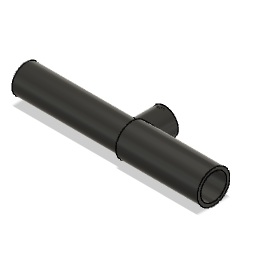
Assemblage bravabot (Autodesk Fusion 360 archive; units mm, degrees)
design "Canon"
Autodesk Fusion 360 part; units mm, degrees
(part 1 of 2)
sketch "Sketch1" plane through (0, 0, 0) normal (0, 0, 1) x (1, 0, 0)
  circle A0 centre (0, 0) radius 16.5
  circle A1 centre (0, 0) radius 15.5
  line L0 (-25, -5) -> (25, -5)
  line L1 (25, -5) -> (25, 5)
  line L2 (25, 5) -> (-25, 5)
  line L3 (-25, 5) -> (-25, -5)
  line L4 (-25, -5) -> (25, 5) construction
  line L5 (25, -5) -> (-25, 5) construction
  line L6 (-5, 25) -> (5, 25)
  line L7 (5, 25) -> (5, -25)
  line L8 (5, -25) -> (-5, -25)
  line L9 (-5, -25) -> (-5, 25)
  line L10 (-5, 25) -> (5, -25) construction
  line L11 (5, 25) -> (-5, -25) construction
  circle A2 centre (0, 4) radius 1
  circle A3 centre (0, -4) radius 1
  circle A4 centre (-3, 0) radius 1
  circle A5 centre (3, 0) radius 1
  dimension "d1" = 33
  dimension "d15" = 31
  dimension "d18" = 50
  dimension "d19" = 10
  dimension "d20" = 10
  dimension "d21" = 50
  dimension "d22" = 2
  dimension "d23" = 2
  dimension "d25" = 2
  dimension "d26" = 4
  dimension "d27" = 8
  dimension "d28" = 2
  dimension "d29" = 3
  dimension "d30" = 6
  constraint coincident A0.centre A1.centre
  constraint horizontal L0
  constraint perpendicular L0 L1
  constraint parallel L0 L2
  constraint parallel L1 L3
  constraint coincident L4 A0.centre
  constraint coincident L5 A0.centre
  constraint horizontal L6
  constraint perpendicular L6 L7
  constraint parallel L6 L8
  constraint parallel L7 L9
  constraint coincident L10 A0.centre
  constraint coincident L11 A0.centre
  measures "d1" diameter of A0
  measures "d15" diameter of A1
  measures "d18" distance of L1.end L2.end
  measures "d19" distance of L0.end L1.end
  measures "d20" distance of L7.end L8.end
  measures "d21" distance of L6.end L7.end
  measures "d22" diameter of A2
  measures "d23" diameter of A3
  measures "d25" diameter of A4
  measures "d26" distance of A0.centre A3.centre
  measures "d27" distance of A2.centre A3.centre
  measures "d28" diameter of A5
  measures "d29" distance of A0.centre A5.centre
  measures "d30" distance of A4.centre A5.centre
extrude "Extrude1" add sketch "Sketch1" along normal blind 37 contours A0 A1 L0 L2 | A0 A1 L2 L7 | A0 A1 L0 L7 | A0 A1 L7 L9 | A1 L2 L7 | A1 L0 L2 L7 | A0 A1 L7 L9 | A1 L0 L7 | A0 A1 L2 L9 | A1 L2 L7 L9 | A2 | A3 | L0 L2 L7 L9 | A0 A1 L0 L9 | A1 L0 L7 L9 | A0 A1 L0 L2 | A1 L2 L9 | A1 L0 L9 | A1 L0 L2 L9 | A4 | A5
sketch "Sketch2" plane through (0, 0, 0) normal (1, 0, 0) x (0, 0, -1)
  circle A0 centre (-39.9957, 0.4126) radius 20
  circle A1 centre (-39.9957, 0.4126) radius 17.5
  circle A2 centre (-39.9957, 0.4126) radius 16
  dimension "d4" = 40
  dimension "d7" = 35
  dimension "d10" = 32
  constraint concentric A0 A1
  constraint concentric A1 A2
  measures "d4" diameter of A0
  measures "d7" diameter of A1
  measures "d10" diameter of A2
extrude "Extrude2" add sketch "Sketch2" along normal blind 100 contours A0 | A1 | A2
extrude "Extrude3" add sketch "Sketch2" against normal blind 130 contours A1 | A2
extrude "Extrude4" cut sketch "Sketch2" along normal blind 140 and the other way blind 90 contours A2
extrude "Extrude5" cut sketch "Sketch1" along normal blind 40 contours A1 L2 L7 | A1 L0 L2 L7 | A1 L0 L7 | A1 L2 L7 L9 | A2 | A3 | L0 L2 L7 L9 | A1 L0 L7 L9 | A1 L2 L9 | A1 L0 L9 | A1 L0 L2 L9 | A4 | A5
extrude "Extrude6" add sketch "Sketch1" along normal blind 2 from surface at 3 contours A1 L0 L2 L7 | A1 L2 L7 L9 | L0 L2 L7 L9 | A1 L0 L7 L9 | A1 L0 L2 L9

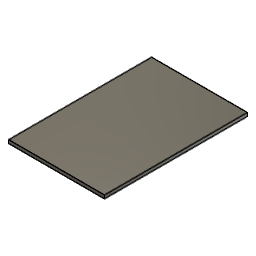
design "Raspberry"
Autodesk Fusion 360 part; units mm, degrees
sketch "Sketch1" plane through (0, 0, 0) normal (0, 1, 0) x (1, 0, 0)
  line L0 (-23.8395, 24.7876) -> (33.1605, 24.7876)
  line L1 (33.1605, 24.7876) -> (33.1605, -60.2124)
  line L2 (33.1605, -60.2124) -> (-23.8395, -60.2124)
  line L3 (-23.8395, -60.2124) -> (-23.8395, 24.7876)
  dimension "d1" = 57
  dimension "d2" = 85
  constraint horizontal L0
  constraint vertical L1
  constraint horizontal L2
  constraint vertical L3
  measures "d1" distance of L0.start L0.end
  measures "d2" distance of L0.start L2.end
extrude "Extrude1" add sketch "Sketch1" along normal blind 2

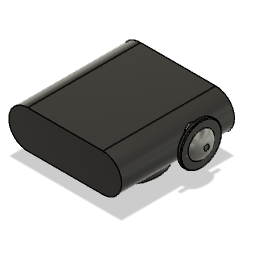
design "tete"
Autodesk Fusion 360 part; units mm, degrees
sketch "Sketch1" plane through (0, 0, 0) normal (0, 0, 1) x (1, 0, 0)
  line L0 (50, 50) -> (0, 50)
  line L1 (0, 50) -> (0, 48)
  arc A0 (50, 0) -> (50, 50) centre (50, 25) ccw
  line L2 (0, 48) -> (48, 48)
  arc A1 (50, 2.0871) -> (48, 48) centre (48, 25) ccw
  arc A2 (-48, 48) -> (-50, 2.0871) centre (-48, 25) ccw
  line L3 (0, 50) -> (0, 48)
  line L4 (-50, 50) -> (0, 50)
  arc A3 (-50, 50) -> (-50, 0) centre (-50, 25) ccw
  line L5 (0, 48) -> (-48, 48)
  line L6 (100, -50) -> (-100, -50)
  line L7 (-100, -50) -> (-100, 100)
  line L8 (-100, 100) -> (100, 100)
  line L9 (100, 100) -> (100, -50)
  line L10 (30.6667, 48) -> (33.3333, 50) construction
  line L11 (-50, 2.0871) -> (-50, 0)
  line L12 (50, 2.0871) -> (50, 0)
  line L13 (-30.6667, 48) -> (-33.3333, 50) construction
  line L14 (-50, 2.0871) -> (50, 2.0871)
  dimension "d1" = 50
  dimension "d2" = 50
  dimension "d8" = 46
  dimension "d9" = 200
  dimension "d10" = 150
  constraint horizontal L0
  constraint vertical L1
  constraint tangent L0 A0
  constraint symmetric A0.start L1 A3.end
  constraint symmetric L0.start L1 L4.start
  constraint symmetric L0.end L1 L3.start
  constraint symmetric L1 A0 A3
  constraint symmetric L1 L2.end A2.start
  constraint symmetric L1 A1 A2
  constraint horizontal L6
  constraint perpendicular L6 L7
  constraint parallel L6 L8
  constraint parallel L7 L9
  constraint vertical L11
  constraint parallel L7 L12
  constraint coincident L2 L10.start
  constraint coincident L5 L13.start
  constraint coincident L0 L10.end
  constraint coincident L4 L13.end
  measures "d1" distance of origin A0.start
  measures "d2" distance of origin L0.end
  measures "d8" diameter of A1
  measures "d9" distance of L7.end L8.end
  measures "d10" distance of L6.end L7.end
extrude "Extrude1" add sketch "Sketch1" along normal blind 146 contours L0 L1 A0 L2 A1 L3 L12 | L1 A2 L3 L4 A3 L5 L11 makes body 1
sketch "Sketch2" plane through (0, 50, 0) normal (0, 1, 0) x (-1, 0, 0)
  line L0 (-50, 0) -> (50, 0)
  line L1 (50, 0) -> (50, 146)
  line L2 (50, 146) -> (-50, 146)
  line L3 (-50, 146) -> (-50, 0)
  line L4 (75, 0) -> (-75, 0)
  line L5 (-75, 0) -> (-75, -2)
  line L6 (-75, -2) -> (75, -2)
  line L7 (75, -2) -> (75, 0)
  line L8 (75, 146) -> (-75, 146)
  line L9 (-75, 146) -> (-75, 148)
  line L10 (-75, 148) -> (75, 148)
  line L11 (75, 148) -> (75, 146)
  dimension "d13" = 150
  dimension "d14" = 2
  dimension "d15" = 150
  dimension "d16" = 2
  constraint horizontal L4
  constraint vertical L5
  constraint horizontal L6
  constraint vertical L7
  constraint horizontal L8
  constraint vertical L9
  constraint horizontal L10
  constraint vertical L11
  measures "d13" distance of L4.start L4.end
  measures "d14" distance of L4.start L6.end
  measures "d15" distance of L8.start L8.end
  measures "d16" distance of L8.start L10.end
extrude "Extrude2" add sketch "Sketch2" against normal blind 70 contours L0 L4 L5 L6 L7 | L2 L8 L9 L10 L11 bodies 1
extrude "Extrude3" cut sketch "Sketch1" along normal blind 150 and the other way blind 50 bodies 1
sketch "Sketch3" plane through (0, 2.0871, 0) normal (0, -1, 0) x (1, 0, 0)
  line L0 (50, 148) -> (-50, 148)
  line L1 (-50, 148) -> (-50, 146)
  line L2 (-50, 146) -> (50, 146)
  line L3 (50, 146) -> (50, 148)
  circle A0 centre (0, 73) radius 48
  circle A1 centre (0, 73) radius 46
  line L4 (-50, 148) -> (50, 148)
  line L5 (50, 148) -> (50, -2)
  line L6 (50, -2) -> (-50, -2)
  line L7 (-50, -2) -> (-50, 148)
  line L8 (-5, 15) -> (5, 15)
  line L9 (5, 15) -> (5, 131)
  line L10 (5, 131) -> (-5, 131)
  line L11 (-5, 131) -> (-5, 15)
  line L12 (-5, 15) -> (5, 131) construction
  line L13 (5, 15) -> (-5, 131) construction
  line L14 (58, 78) -> (-58, 78)
  line L15 (-58, 78) -> (-58, 68)
  line L16 (-58, 68) -> (58, 68)
  line L17 (58, 68) -> (58, 78)
  line L18 (58, 78) -> (-58, 68) construction
  line L19 (-58, 78) -> (58, 68) construction
  circle A2 centre (0, 67) radius 1
  circle A3 centre (4, 73) radius 1
  circle A4 centre (-4, 73) radius 1
  circle A5 centre (0, 79) radius 1
  point P0 (0, 73)
  point P1 (0, 73)
  dimension "d23" = 96
  dimension "d24" = 75
  dimension "d25" = 92
  dimension "d33" = 116
  dimension "d34" = 10
  dimension "d35" = 2
  dimension "d36" = 2
  dimension "d37" = 2
  dimension "d38" = 2
  dimension "d39" = 12
  dimension "d40" = 6
  dimension "d41" = 4
  dimension "d42" = 8
  constraint concentric A0 A1
  constraint horizontal L4
  constraint vertical L5
  constraint horizontal L6
  constraint vertical L7
  constraint coincident L0.end L1.start
  constraint horizontal L8
  constraint perpendicular L8 L9
  constraint parallel L8 L10
  constraint parallel L9 L11
  constraint coincident L12 P1
  constraint coincident L13 P1
  constraint coincident P1 P0
  constraint horizontal L14
  constraint perpendicular L14 L15
  constraint parallel L14 L16
  constraint parallel L15 L17
  constraint coincident L18 P1
  constraint coincident L19 P1
  measures "d23" diameter of A0
  measures "d24" distance of L0 P1
  measures "d25" diameter of A1
  measures "d33" distance of L15.end L16.end
  measures "d34" distance of L14.end L15.end
  measures "d35" diameter of A2
  measures "d36" diameter of A3
  measures "d37" diameter of A4
  measures "d38" diameter of A5
  measures "d39" distance of A2.centre A5.centre
  measures "d40" distance of P1 A2.centre
  measures "d41" distance of P1 A4.centre
  measures "d42" distance of A3.centre A4.centre
extrude "Extrude4" add sketch "Sketch3" along normal blind 2 contours L0 L1 L2 L3 L4 L5 L7 | L2 A0 L5 L7 L9 L10 L11 L14 | A0 L5 L14 L16 | A0 L7 L14 L16 | A0 L5 L6 L7 L8 L9 L11 L16 | A0 L9 L10 L11 | A0 L8 L9 L11 bodies 1
extrude "Extrude5" add sketch "Sketch3" along normal blind 20 contours A0 A1 L9 L14 | A0 A1 L14 L16 | A0 A1 L14 L16 | A0 A1 L11 L14 | A0 A1 L9 L16 | A0 A1 L9 L11 | A0 A1 L11 L16 | A0 A1 L9 L11 bodies 1
sketch "Sketch4" plane through (0, 0, -2) normal (0, 0, -1) x (-1, 0, 0)
  arc A0 (-50, 50) -> (-50, 0) centre (-50, 25) ccw
  line L0 (-50, 0) -> (-50, 0.0871)
  line L1 (-50, 0.0871) -> (50, 0.0871)
  line L2 (50, 0.0871) -> (50, 0)
  arc A1 (50, 0) -> (50, 50) centre (50, 25) ccw
  line L3 (50, 50) -> (-50, 50)
  circle A2 centre (0, 25) radius 17.5
  line L4 (20, 20) -> (-20, 20)
  line L5 (-20, 20) -> (-20, 30)
  line L6 (-20, 30) -> (20, 30)
  line L7 (20, 30) -> (20, 20)
  line L8 (20, 20) -> (-20, 30) construction
  line L9 (-20, 20) -> (20, 30) construction
  line L10 (-6.6445, 5) -> (6.6445, 5)
  line L11 (6.6445, 5) -> (6.6445, 45)
  line L12 (6.6445, 45) -> (-6.6445, 45)
  line L13 (-6.6445, 45) -> (-6.6445, 5)
  line L14 (-6.6445, 5) -> (6.6445, 45) construction
  line L15 (6.6445, 5) -> (-6.6445, 45) construction
  line L16 (13.5, 19) -> (-13.5, 19)
  line L17 (-13.5, 19) -> (-13.5, 31)
  line L18 (-13.5, 31) -> (13.5, 31)
  line L19 (13.5, 31) -> (13.5, 19)
  line L20 (13.5, 19) -> (-13.5, 31) construction
  line L21 (-13.5, 19) -> (13.5, 31) construction
  line L22 (14.5, 18) -> (-14.5, 18)
  line L23 (-14.5, 18) -> (-14.5, 32)
  line L24 (-14.5, 32) -> (14.5, 32)
  line L25 (14.5, 32) -> (14.5, 18)
  line L26 (14.5, 18) -> (-14.5, 32) construction
  line L27 (-14.5, 18) -> (14.5, 32) construction
  point P0 (0, 25)
  point P1 (0, 25)
  point P2 (0, 25)
  point P3 (0, 25)
  dimension "d30" = 35
  dimension "d45" = 40
  dimension "d46" = 10
  dimension "d47" = 40
  dimension "d48" = 27
  dimension "d49" = 12
  dimension "d50" = 29
  dimension "d51" = 14
  constraint horizontal L4
  constraint perpendicular L4 L5
  constraint parallel L4 L6
  constraint parallel L5 L7
  constraint coincident L8 P3
  constraint coincident L9 P3
  constraint coincident P3 P2
  constraint horizontal L10
  constraint perpendicular L10 L11
  constraint parallel L10 L12
  constraint parallel L11 L13
  constraint coincident L14 P3
  constraint coincident L15 P3
  constraint horizontal L16
  constraint perpendicular L16 L17
  constraint parallel L16 L18
  constraint parallel L17 L19
  constraint coincident L20 P3
  constraint coincident L21 P3
  constraint horizontal L22
  constraint perpendicular L22 L23
  constraint parallel L22 L24
  constraint parallel L23 L25
  constraint coincident L26 P3
  constraint coincident L27 P3
  measures "d30" diameter of A2
  measures "d45" distance of L5.end L6.end
  measures "d46" distance of L4.end L5.end
  measures "d47" distance of L10.end L11.end
  measures "d48" distance of L17.end L18.end
  measures "d49" distance of L16.end L17.end
  measures "d50" distance of L23.end L24.end
  measures "d51" distance of L22.end L23.end
extrude "Extrude6" cut sketch "Sketch4" against normal blind 20 contours A2 L4 L6 L25 | A2 L6 L11 L24 L25 | A2 L4 L11 L22 L25 | A2 L11 L13 L24 | L4 L6 L19 L25 | L6 L11 L18 L19 L24 L25 | A2 L11 L13 L22 | L4 L11 L16 L19 L22 L25 | A2 L6 L13 L23 L24 | L11 L13 L18 L24 | L4 L6 L11 L19 | L6 L11 L18 L19 | A2 L4 L13 L22 L23 | L11 L13 L16 L22 | L4 L11 L16 L19 | A2 L4 L6 L23 | L6 L13 L17 L18 L23 L24 | L6 L11 L13 L18 | L4 L6 L11 L13 | L4 L13 L16 L17 L22 L23 | L4 L11 L13 L16 | L4 L6 L17 L23 | L6 L13 L17 L18 | L4 L6 L13 L17 | L4 L13 L16 L17 bodies 1
extrude "Extrude7" add sketch "Sketch3" along normal blind 3 contours A1 L9 L14 L16 | A1 L11 L14 L16 | A1 L9 L11 L14 | L9 L11 L14 L16 | A1 L9 L11 L16 bodies 1
extrude "Extrude8" add sketch "Sketch4" against normal blind 9 contours A2 L4 L6 L7 | A2 L11 L12 L13 | A2 L10 L11 L13 | A2 L4 L5 L6 bodies 1
extrude "Extrude9" add sketch "Sketch4" along normal blind 2 and the other way blind 15 separate body contours L4 L6 L19 L25 | L6 L11 L18 L19 L24 L25 | L4 L11 L16 L19 L22 L25 | L11 L13 L18 L24 | L11 L13 L16 L22 | L6 L13 L17 L18 L23 L24 | L4 L13 L16 L17 L22 L23 | L4 L6 L17 L23 makes body 2
extrude "Extrude10" add sketch "Sketch4" against normal blind 3 from surface at -6 separate body contours A2 L4 L6 L25 | A2 L11 L13 L24 | A2 L11 L13 L22 | A2 L4 L6 L23 makes body 3 at (0, 14.5, 4) makes body 4 at (0, 35.5, 4) makes body 5 at (16.9923, 20.8154, 6) makes body 6 at (-17.4184, 23.3124, 5)
ref_plane "WorkPlane1" through (75, 0, 0) normal (1, 0, 0) x (0, 1, 0)
sketch "Sketch6" plane through (75, 0, 0) normal (1, 0, 0) x (0, 0, -1)
  circle A0 centre (-50, 25) radius 17.5
  circle A1 centre (-50, 25) radius 27.5
  dimension "d62" = 35
  dimension "d63" = 55
  constraint concentric A0 A1
  measures "d62" diameter of A0
  measures "d63" diameter of A1
extrude "Extrude11" add sketch "Sketch6" along normal blind 15 and the other way blind 10 contours A0 bodies 1 6 5 4 3 2
extrude "Extrude12" add sketch "Sketch6" along normal blind 5 from surface at 3 bodies 1 2 3 6 5 4
fillet "Fillet1" radius 17.5 1 edges at (90, 18.6717, 66.3157) on bodies 1
fillet "Fillet2" radius 1 2 edges at (83, 15.0556, 75.639) (78, 15.0556, 75.639) on bodies 1

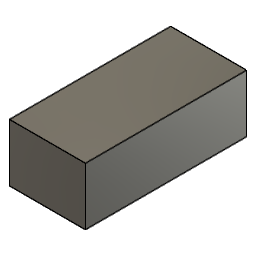
design "Batterie"
Autodesk Fusion 360 part; units mm, degrees
sketch "Sketch1" plane through (0, 0, 0) normal (0, 1, 0) x (1, 0, 0)
  line L0 (-8, 7) -> (-41, 7)
  line L1 (-41, 7) -> (-41, -63)
  line L2 (-41, -63) -> (-8, -63)
  line L3 (-8, -63) -> (-8, 7)
  dimension "d1" = 33
  dimension "d2" = 70
  constraint horizontal L0
  constraint vertical L1
  constraint horizontal L2
  constraint vertical L3
  measures "d1" distance of L0.start L0.end
  measures "d2" distance of L0.start L2.end
extrude "Extrude1" add sketch "Sketch1" along normal blind 25

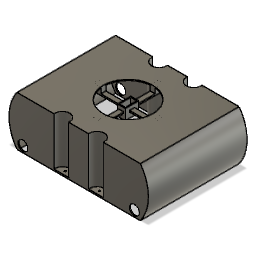
design "Carter BravaBot"
Autodesk Fusion 360 part; units mm, degrees
sketch "Sketch1" plane through (0, 0, 0) normal (0, 0, 1) x (1, 0, 0)
  line L0 (0, 0) -> (-125, 0)
  line L1 (-125, 100) -> (0, 100)
  line L2 (0, 100) -> (0, 0)
  arc A0 (-125, 100) -> (-125, 0) centre (-56.2614, 50) ccw
  arc A1 (-124.4112, 98) -> (-123, 0) centre (-54.2614, 50) ccw
  line L3 (0, 98) -> (-124.4112, 98)
  line L4 (-175, 98) -> (-175, -10)
  line L5 (-175, -10) -> (191.1619, -10)
  line L6 (191.1619, -10) -> (191.1619, 126.0853)
  line L7 (191.1619, 126.0853) -> (-175, 126.0853)
  line L8 (-175, 126.0853) -> (-175, 98)
  line L9 (0, 98) -> (124.4112, 98)
  line L10 (125, 100) -> (0, 100)
  arc A2 (123, 0) -> (124.4112, 98) centre (54.2614, 50) ccw
  arc A3 (125, 0) -> (125, 100) centre (56.2614, 50) ccw
  line L11 (0, 0) -> (125, 0)
  circle A4 centre (113, 12.5) radius 10
  circle A5 centre (-113, 12.5) radius 10
  dimension "d1" = 125
  dimension "d2" = 100
  dimension "d3" = 85
  dimension "d4" = 85
  dimension "d6" = 2
  dimension "d7" = 2
  dimension "d44" = 20
  dimension "d45" = 12
  dimension "d46" = 12.5
  constraint horizontal L0
  constraint horizontal L1
  constraint vertical L2
  constraint coincident L0.start L2.end
  constraint coincident L0 A1.end
  constraint coincident L2 L3.start
  constraint perpendicular L2 L3
  constraint perpendicular L3 L4
  constraint perpendicular L4 L5
  constraint perpendicular L5 L6
  constraint perpendicular L6 L7
  constraint perpendicular L3 L8
  constraint symmetric L0.start L2 L11.start
  constraint symmetric L0.end L2 A3.start
  constraint symmetric L1.start L2 L10.start
  constraint symmetric L1.end L2 L10.end
  constraint symmetric L2 A0 A3
  constraint symmetric L2 A1.end A2.start
  constraint symmetric L2 A1 A2
  constraint symmetric L2 L3.start L9.start
  constraint symmetric L2 A1.start L9.end
  constraint symmetric L2 A4 A5
  measures "d1" distance of L0.start L0.end
  measures "d2" distance of L0.start L1.end
  measures "d3" radius of A0
  measures "d4" radius of A1
  measures "d6" distance of L0.end A1.end
  measures "d7" distance of L1 L3
  measures "d44" diameter of A4
  measures "d45" horizontal distance of A3.start A4.centre
  measures "d46" distance of L11 A4.centre
extrude "Extrude1" add sketch "Sketch1" along normal blind 196 contours L0 L1 L2 A0 A1 L3 | L2 L9 L10 A2 A3 L11 makes body 1
sketch "Sketch2" plane through (0, 100, 0) normal (0, 1, 0) x (-1, 0, 0)
  line L0 (-125, 0) -> (125, 0)
  line L1 (125, 0) -> (125, 196)
  line L2 (125, 196) -> (-125, 196)
  line L3 (-125, 196) -> (-125, 0)
  line L4 (56.5763, 0) -> (165.4437, 0)
  line L5 (165.4437, 0) -> (165.4437, -2)
  line L6 (165.4437, -2) -> (56.5763, -2)
  line L7 (56.5763, -2.1497) -> (56.5763, -2)
  line L8 (27.1632, 196) -> (155, 196)
  line L9 (155, 196) -> (155, 198)
  line L10 (155, 198) -> (27.1632, 198)
  line L11 (27.1632, 196) -> (-160, 196)
  line L12 (-160, 196) -> (-160, 198)
  line L13 (-160, 198) -> (27.1632, 198)
  line L14 (56.5763, 0) -> (-160, 0)
  line L15 (-160, 0) -> (-160, -2)
  line L16 (-160, -2) -> (56.5763, -2)
  line L17 (56.5763, -2) -> (56.5763, 0)
  circle A0 centre (-35, 196) radius 15
  circle A1 centre (-35, 196) radius 17
  circle A2 centre (35, 196) radius 15
  circle A3 centre (35, 196) radius 17
  circle A4 centre (-35, 0) radius 17
  circle A5 centre (-35, 0) radius 15
  circle A6 centre (35, 0) radius 17
  circle A7 centre (35, 0) radius 15
  circle A8 centre (-35, 6) radius 2
  circle A9 centre (35, 6) radius 2
  line L18 (-50, 0) -> (-50, 25)
  line L19 (20, 0) -> (20, 24.2158)
  circle A10 centre (35, 190) radius 2
  circle A11 centre (-35, 190) radius 2
  circle A12 centre (0, 98) radius 50
  line L20 (65, 103) -> (65, 93)
  line L21 (-65, 93) -> (-65, 103)
  line L22 (-5, 33) -> (5, 33)
  line L23 (5, 163) -> (-5, 163)
  line L24 (-6, 109.5) -> (6, 109.5)
  line L25 (6, 86.5) -> (-6, 86.5)
  line L26 (-8, 93) -> (-65, 93)
  line L27 (65, 93) -> (8, 93)
  line L28 (5, 33) -> (5, 84.5)
  line L29 (5, 111.5) -> (5, 163)
  line L30 (65, 103) -> (8, 98.6154) construction
  line L31 (-8, 97.3846) -> (-65, 93) construction
  line L32 (-65, 103) -> (-8, 98.6154) construction
  line L33 (8, 97.3846) -> (65, 93) construction
  line L34 (-125, 98) -> (-8, 98)
  line L35 (8, 98) -> (125, 98)
  line L36 (-5, 33) -> (-1.0385, 84.5) construction
  line L37 (1.0385, 111.5) -> (5, 163) construction
  line L38 (5, 33) -> (1.0385, 84.5) construction
  line L39 (-1.0385, 111.5) -> (-5, 163) construction
  line L40 (-65, 103) -> (-8, 103)
  line L41 (8, 103) -> (65, 103)
  line L42 (-5, 84.5) -> (-5, 33)
  line L43 (-5, 163) -> (-5, 111.5)
  line L44 (6, 109.5) -> (6, 98)
  line L45 (6, 97.5385) -> (6, 86.5)
  line L46 (-6, 86.5) -> (-6, 98.4615)
  line L47 (-6, 103) -> (-6, 109.5)
  line L48 (-6, 103) -> (-6, 98.4615)
  line L49 (-8, 84.5) -> (8, 84.5)
  line L50 (8, 84.5) -> (8, 111.5)
  line L51 (8, 111.5) -> (-8, 111.5)
  line L52 (-8, 111.5) -> (-8, 84.5)
  line L53 (6, 98) -> (6, 97.5385)
  point P0 (0, 98)
  point P1 (0, 98)
  point P2 (0, 98)
  point P3 (0, 98)
  dimension "d10" = 2
  dimension "d11" = 2
  dimension "d12" = 2
  dimension "d15" = 2
  dimension "d22" = 30
  dimension "d23" = 34
  dimension "d24" = 30
  dimension "d25" = 34
  dimension "d26" = 90
  dimension "d27" = 90
  dimension "d35" = 4
  dimension "d36" = 4
  dimension "d37" = 15
  dimension "d38" = 15
  dimension "d39" = 6
  dimension "d40" = 6
  dimension "d41" = 100
  dimension "d55" = 130
  dimension "d56" = 10
  dimension "d57" = 10
  dimension "d58" = 130
  dimension "d59" = 12
  dimension "d60" = 23
  dimension "d61" = 16
  dimension "d62" = 27
  constraint perpendicular L4 L5
  constraint parallel L4 L6
  constraint perpendicular L1 L4
  constraint coincident L0 L4.start
  constraint vertical L7
  constraint horizontal L8
  constraint vertical L9
  constraint horizontal L10
  constraint coincident L2 L8.start
  constraint horizontal L11
  constraint vertical L12
  constraint horizontal L13
  constraint horizontal L14
  constraint vertical L15
  constraint horizontal L16
  constraint vertical L17
  constraint concentric A0 A1
  constraint concentric A2 A3
  constraint midpoint L3 L34.start
  constraint midpoint L1 L35.end
  constraint coincident L8 A2.centre
  constraint coincident L11 A0.centre
  constraint symmetric A0 A5 L34
  constraint symmetric A1 A4 L34
  constraint symmetric A2 A7 L34
  constraint symmetric A3 A6 L34
  constraint coincident A5 L18.start
  constraint coincident L14 L18.start
  constraint tangent A5 L18
  constraint coincident A7 L19.start
  constraint coincident L14 L19.start
  constraint tangent A7 L19
  constraint symmetric A8 A11 L34
  constraint symmetric A9 A10 L34
  constraint horizontal L40
  constraint perpendicular L20 L40
  constraint parallel L27 L40
  constraint parallel L20 L21
  constraint coincident P3 L32
  constraint coincident P3 L30
  constraint coincident P3 P2
  constraint horizontal L22
  constraint perpendicular L22 L28
  constraint parallel L22 L23
  constraint parallel L28 L43
  constraint coincident P3 L36
  constraint coincident P3 L38
  constraint horizontal L24
  constraint perpendicular L24 L44
  constraint parallel L24 L25
  constraint parallel L44 L46
  constraint collinear L26 L27
  constraint collinear L30 L31
  constraint collinear L32 L33
  constraint collinear L34 L35
  constraint collinear L36 L37
  constraint collinear L38 L39
  constraint collinear L40 L41
  constraint collinear L42 L43
  constraint coincident L47.start L46
  constraint coincident L45.start L44
  constraint collinear L44 L45
  constraint collinear L46 L47
  constraint horizontal L49
  constraint perpendicular L49 L50
  constraint parallel L49 L51
  constraint parallel L50 L52
  constraint coincident L49 L28.end
  constraint coincident L50 L27.end
  constraint coincident L50 L35.start
  constraint coincident L50 L33.start
  constraint coincident L50 L30.end
  constraint coincident L50 L41.start
  constraint coincident L52 L34.end
  constraint coincident L52 L32.end
  constraint coincident L52 L31.start
  constraint coincident L52 L26.start
  constraint coincident L49 L42.start
  constraint coincident L49 L36.end
  constraint coincident L49 L38.end
  constraint coincident L52 L40.end
  constraint coincident L51 L43.end
  constraint coincident L51 L29.start
  constraint coincident L51 L37.start
  constraint coincident L51 L39.start
  measures "d10" distance of L8 L10
  measures "d11" distance of L11 L13
  measures "d12" distance of L4 L6
  measures "d15" distance of L4.start L6.end
  measures "d22" diameter of A0
  measures "d23" diameter of A1
  measures "d24" diameter of A2
  measures "d25" diameter of A3
  measures "d26" distance of L3 A0.centre
  measures "d27" distance of L1 A2.centre
  measures "d35" diameter of A8
  measures "d36" diameter of A9
  measures "d37" distance of A8.centre L18
  measures "d38" distance of A9.centre L19
  measures "d39" distance of L14 A8.centre
  measures "d40" distance of L14 A9.centre
  measures "d41" diameter of A12
  measures "d55" distance of L20.end L21.start
  measures "d56" distance of L27 L40
  measures "d57" distance of L23.start L23.end
  measures "d58" distance of L22.end L23.start
  measures "d59" distance of L25.start L25.end
  measures "d60" distance of L24.end L25.start
  measures "d61" distance of L50.end L51.end
  measures "d62" distance of L49.end L50.end
extrude "Extrude2" add sketch "Sketch2" against normal blind 100 contours L0 L14 L16 A4 A5 | L0 L14 L16 A5 | L0 L14 L16 A4 A5 | L0 L14 L15 L16 A4 | L0 L14 L16 A4 A6 | L0 L14 L16 A6 A7 | L0 L14 L16 A7 | L2 L11 L12 L13 A1 | L0 L14 L16 A6 A7 | L0 L14 L16 L17 A6 | L2 L11 L13 A0 A1 | L0 L4 L5 L6 L17 | L2 L11 L13 A0 | L2 L11 L13 A1 A3 | L2 L11 L13 A0 A1 | L2 L11 L13 A2 A3 | L2 L8 L10 L11 L13 A2 | L2 L8 L9 L10 A3 | L2 L8 L10 A2 A3 bodies 1
extrude "Extrude3" cut sketch "Sketch1" along normal blind 270 and the other way blind 120 contours L4 L5 L6 L7 L8 bodies 1
extrude "Extrude4" cut sketch "Sketch2" against normal blind 120 contours L0 L14 A5 | L0 L14 L16 A5 | L0 L14 A7 | L0 L14 L16 A7 | L2 L11 L13 A0 | L2 L11 A0 | L2 L8 L10 L11 L13 A2 | L2 L8 L11 A2 | A8 | A9 | A10 | A11 bodies 1
extrude "Extrude5" add sketch "Sketch2" against normal blind 100 contours L0 L14 L16 A4 A5 | L0 L14 A4 A5 L18 | L0 L14 A4 L18 | L0 L14 L16 A4 A5 | L0 L14 A6 L19 | L0 L14 L16 A6 A7 | L0 L14 A6 A7 L19 | L0 L14 L16 A6 A7 | L2 L11 L13 A0 A1 | L2 L11 A0 A1 | L2 L11 L13 A0 A1 | L2 L11 L13 A2 A3 | L2 L8 L11 A2 A3 | L2 L8 L10 A2 A3 bodies 1
extrude "Extrude6" add sketch "Sketch2" against normal blind 3 from surface at -97 contours L0 L14 A5 | L0 L14 L16 A5 | L0 L14 A7 | L0 L14 L16 A7 | L2 L11 L13 A0 | L2 L11 A0 | L2 L8 L10 L11 L13 A2 | L2 L8 L11 A2 | A8 | A9 | A10 | A11 bodies 1
extrude "Extrude7" cut sketch "Sketch2" against normal blind 180 contours A12 L26 L34 L52 | A12 L34 L40 L52 | A12 L26 L42 L49 L52 | A12 L40 L43 L51 L52 | L49 L50 L51 L52 | A12 L28 L42 L49 | A12 L29 L43 L51 | A12 L27 L28 L49 L50 | A12 L29 L41 L50 L51 | A12 L27 L35 L50 | A12 L35 L41 L50 | A8 | A9 | A10 | A11 | L24 L25 L44 L45 L46 L47 L48 L53 bodies 1
extrude "Extrude8" cut sketch "Sketch1" along normal blind 250 and the other way blind 25 contours A4 | A5 bodies 1
extrude "Extrude9" add sketch "Sketch2" against normal blind 3 from surface at -12.5 separate body contours A12 L26 L34 L52 | A12 L34 L40 L52 | A12 L28 L42 L49 | A12 L29 L43 L51 | A12 L27 L35 L50 | A12 L35 L41 L50 makes body 2 at (0.5564, 87.5, 123.6574) makes body 3 at (21.9907, 84.5, 98.5564) makes body 4 at (-21.9907, 84.5, 98.5564) makes body 5 at (0.5564, 87.5, 72.3426)
extrude "Extrude10" add sketch "Sketch2" against normal blind 21.5 from surface at -5 contours L49 L50 L51 L52 bodies 2 3 4 5
extrude "Extrude11" add sketch "Sketch2" against normal blind 2 from surface at -24.5 contours L24 L25 L44 L45 L46 L47 L48 L53 bodies 2
extrude "Extrude12" add sketch "Sketch2" against normal blind 15.5 contours A12 L21 L26 L34 | A12 L21 L34 L40 | A12 L22 L28 L42 | A12 L23 L29 L43 | A12 L20 L35 L41 | A12 L20 L27 L35 bodies 1 2
sketch "Sketch3" plane through (0, 0, 86.5) normal (0, 0, 1) x (1, 0, 0)
  line L0 (-6, 75.5) -> (6, 75.5)
  line L1 (6, 75.5) -> (6, 95)
  line L2 (6, 95) -> (-6, 95)
  line L3 (-6, 95) -> (-6, 75.5)
  line L4 (-5, 77) -> (5, 77)
  line L5 (5, 77) -> (5, 84.4286)
  line L6 (5, 84.4286) -> (-5, 84.4286)
  line L7 (-5, 84.4286) -> (-5, 77)
  constraint horizontal L4
  constraint vertical L5
  constraint horizontal L6
  constraint vertical L7
extrude "Extrude13" cut sketch "Sketch3" against normal blind 2 contours L4 L5 L6 L7 bodies 1

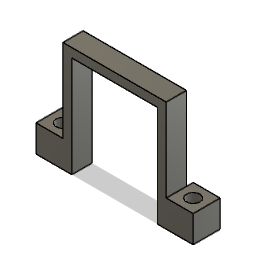
design "fixation moto-réducteur"
Autodesk Fusion 360 part; units mm, degrees
sketch "Sketch1" plane through (0, 0, 0) normal (0, 0, 1) x (1, 0, 0)
  line L0 (0, 0) -> (6, 0)
  line L1 (6, 0) -> (6, 6)
  line L2 (6, 6) -> (0, 6)
  line L3 (0, 6) -> (0, 0)
  line L4 (6, 0) -> (8, 0)
  line L5 (8, 0) -> (8, 24.5)
  line L6 (8, 24.5) -> (6, 24.5)
  line L7 (6, 24.5) -> (6, 0)
  line L8 (6, 24.5) -> (17.5, 24.5)
  line L9 (17.5, 24.5) -> (17.5, 22.5)
  line L10 (17.5, 22.5) -> (6, 22.5)
  line L11 (6, 22.5) -> (6, 24.5)
  line L12 (29, 6) -> (35, 6)
  line L13 (17.5, 22.5) -> (29, 22.5)
  line L14 (29, 0) -> (29, 6)
  line L15 (35, 6) -> (35, 0)
  line L16 (29, 24.5) -> (29, 0)
  line L17 (27, 24.5) -> (29, 24.5)
  line L18 (17.5, 24.5) -> (17.5, 22.5)
  line L19 (29, 22.5) -> (29, 24.5)
  line L20 (35, 0) -> (29, 0)
  line L21 (29, 24.5) -> (17.5, 24.5)
  line L22 (27, 0) -> (27, 24.5)
  line L23 (29, 0) -> (27, 0)
  point P0 (35, 0)
  dimension "d1" = 6
  dimension "d2" = 6
  dimension "d3" = 2
  dimension "d4" = 24.5
  dimension "d5" = 11.5
  dimension "d6" = 2
  constraint horizontal L0
  constraint vertical L1
  constraint horizontal L2
  constraint vertical L3
  constraint coincident L0.start L3.end
  constraint horizontal L4
  constraint vertical L5
  constraint horizontal L6
  constraint vertical L7
  constraint horizontal L8
  constraint vertical L9
  constraint horizontal L10
  constraint vertical L11
  constraint symmetric L0.start L9 L15.end
  constraint symmetric L0.start L9 P0
  constraint symmetric L0.end L9 L14.start
  constraint symmetric L1.end L9 L12.start
  constraint symmetric L2.end L9 L12.end
  constraint symmetric L4.end L9 L22.start
  constraint symmetric L5.end L9 L17.start
  constraint symmetric L6.end L9 L16.start
  constraint symmetric L8.end L9 L18.start
  constraint symmetric L10.start L9 L13.start
  constraint symmetric L10.end L9 L13.end
  measures "d1" distance of L0.start L0.end
  measures "d2" distance of L0.start L2.end
  measures "d3" distance of L0.end L4.end
  measures "d4" distance of L0.end L6.end
  measures "d5" distance of L6.end L8.end
  measures "d6" distance of L6.end L10.end
extrude "Extrude1" add sketch "Sketch1" along normal blind 3 and the other way blind 3 contours L0 L1 L2 L3 L7 | L12 L14 L15 L16 L20 makes body 1 at (31, 6, -1) makes body 2 at (0, 2, 1)
extrude "Extrude2" add sketch "Sketch1" along normal blind 1.5 and the other way blind 1.5 contours L1 L4 L5 L7 L10 | L5 L6 L7 L8 L10 L11 | L5 L8 L9 L10 L18 | L9 L13 L18 L21 L22 | L13 L16 L17 L19 L21 L22 | L13 L14 L16 L22 L23 bodies 1 2
sketch "Sketch3" plane through (0, 6, 0) normal (0, 1, 0) x (-1, 0, 0)
  line L0 (0, -3) -> (0, 3)
  line L1 (0, 3) -> (-6, 3)
  line L2 (-6, 3) -> (-6, 1.5)
  line L3 (-6, 1.5) -> (-6, -1.5)
  line L4 (-6, -1.5) -> (-6, -3)
  line L5 (-6, -3) -> (0, -3)
  circle A0 centre (-3, 0) radius 1.5
  circle A1 centre (-32, 0) radius 1.5
  line L6 (-35, -3) -> (-35, 3)
  line L7 (-29, -3) -> (-35, -3)
  dimension "d16" = 3
  dimension "d17" = 3
  dimension "d18" = 3
  dimension "d19" = 3
  dimension "d20" = 3
  dimension "d21" = 3
  measures "d16" diameter of A0
  measures "d17" diameter of A1
  measures "d18" distance of L5 A0.centre
  measures "d19" distance of L0 A0.centre
  measures "d20" distance of A1.centre L6
  measures "d21" distance of A1.centre L7
extrude "Extrude3" cut sketch "Sketch3" against normal blind 11 contours A0 | A1 bodies 1
extrude "Extrude4" add 1 faces at (27.6667, 9.5, 1.5) along direction (0, 0, 1) up to surface (1.5 mm away) on bodies 1 bodies 1

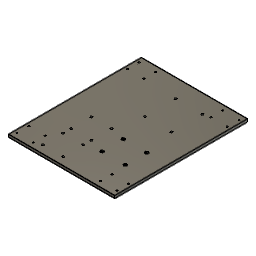
design "base roulante essaie"
Autodesk Fusion 360 part; units mm, degrees
sketch "Sketch1" plane through (0, 0, 0) normal (0, 1, 0) x (1, 0, 0)
  line L0 (0, 0) -> (200, 0)
  line L1 (200, 0) -> (200, 250)
  line L2 (200, 250) -> (0, 250)
  line L3 (0, 250) -> (0, 0)
  circle A0 centre (6, 240) radius 1.5
  circle A1 centre (37, 240) radius 1.5
  line L4 (100, 250) -> (100, 0)
  line L5 (0, 125) -> (200, 125)
  circle A2 centre (163, 240) radius 1.5
  circle A3 centre (194, 240) radius 1.5
  circle A4 centre (6, 10) radius 1.5
  circle A5 centre (163, 10) radius 1.5
  circle A6 centre (37, 10) radius 1.5
  circle A7 centre (194, 10) radius 1.5
  circle A8 centre (6, 218) radius 1.5
  circle A9 centre (37, 218) radius 1.5
  circle A10 centre (163, 218) radius 1.5
  circle A11 centre (194, 218) radius 1.5
  circle A12 centre (37, 32) radius 1.5
  circle A13 centre (6, 32) radius 1.5
  circle A14 centre (194, 32) radius 1.5
  circle A15 centre (163, 32) radius 1.5
  line L6 (34.25, 238.4123) -> (37, 236.8246)
  line L7 (37, 236.8246) -> (39.75, 238.4123)
  line L8 (39.75, 238.4123) -> (39.75, 241.5877)
  line L9 (39.75, 241.5877) -> (37, 243.1754)
  line L10 (37, 243.1754) -> (34.25, 241.5877)
  line L11 (34.25, 241.5877) -> (34.25, 238.4123)
  line L12 (8.75, 238.4123) -> (8.75, 241.5877)
  line L13 (8.75, 241.5877) -> (6, 243.1754)
  line L14 (6, 243.1754) -> (3.25, 241.5877)
  line L15 (3.25, 241.5877) -> (3.25, 238.4123)
  line L16 (3.25, 238.4123) -> (6, 236.8246)
  line L17 (6, 236.8246) -> (8.75, 238.4123)
  line L18 (34.25, 219.5877) -> (34.25, 216.4123)
  line L19 (34.25, 216.4123) -> (37, 214.8246)
  line L20 (37, 214.8246) -> (39.75, 216.4123)
  line L21 (39.75, 216.4123) -> (39.75, 219.5877)
  line L22 (39.75, 219.5877) -> (37, 221.1754)
  line L23 (37, 221.1754) -> (34.25, 219.5877)
  line L24 (3.25, 219.5877) -> (3.25, 216.4123)
  line L25 (3.25, 216.4123) -> (6, 214.8246)
  line L26 (6, 214.8246) -> (8.75, 216.4123)
  line L27 (8.75, 216.4123) -> (8.75, 219.5877)
  line L28 (8.75, 219.5877) -> (6, 221.1754)
  line L29 (6, 221.1754) -> (3.25, 219.5877)
  line L30 (191.25, 238.4123) -> (191.25, 241.5877)
  line L31 (194, 214.8246) -> (191.25, 216.4123)
  line L32 (160.25, 219.5877) -> (163, 221.1754)
  line L33 (163, 214.8246) -> (160.25, 216.4123)
  line L34 (163, 236.8246) -> (160.25, 238.4123)
  line L35 (194, 221.1754) -> (196.75, 219.5877)
  line L36 (191.25, 219.5877) -> (194, 221.1754)
  line L37 (196.75, 219.5877) -> (196.75, 216.4123)
  line L38 (194, 236.8246) -> (191.25, 238.4123)
  line L39 (160.25, 238.4123) -> (160.25, 241.5877)
  line L40 (160.25, 216.4123) -> (160.25, 219.5877)
  line L41 (196.75, 238.4123) -> (194, 236.8246)
  line L42 (196.75, 216.4123) -> (194, 214.8246)
  line L43 (160.25, 241.5877) -> (163, 243.1754)
  line L44 (165.75, 219.5877) -> (165.75, 216.4123)
  line L45 (196.75, 241.5877) -> (196.75, 238.4123)
  line L46 (163, 221.1754) -> (165.75, 219.5877)
  line L47 (165.75, 216.4123) -> (163, 214.8246)
  line L48 (194, 243.1754) -> (196.75, 241.5877)
  line L49 (191.25, 216.4123) -> (191.25, 219.5877)
  line L50 (165.75, 238.4123) -> (163, 236.8246)
  line L51 (191.25, 241.5877) -> (194, 243.1754)
  line L52 (163, 243.1754) -> (165.75, 241.5877)
  line L53 (165.75, 241.5877) -> (165.75, 238.4123)
  line L54 (8.75, 33.5877) -> (8.75, 30.4123)
  line L55 (37, 28.8246) -> (34.25, 30.4123)
  line L56 (34.25, 8.4123) -> (34.25, 11.5877)
  line L57 (37, 35.1754) -> (39.75, 33.5877)
  line L58 (6, 35.1754) -> (8.75, 33.5877)
  line L59 (34.25, 33.5877) -> (37, 35.1754)
  line L60 (37, 6.8246) -> (34.25, 8.4123)
  line L61 (3.25, 8.4123) -> (3.25, 11.5877)
  line L62 (39.75, 11.5877) -> (39.75, 8.4123)
  line L63 (6, 13.1754) -> (8.75, 11.5877)
  line L64 (37, 13.1754) -> (39.75, 11.5877)
  line L65 (39.75, 8.4123) -> (37, 6.8246)
  line L66 (39.75, 30.4123) -> (37, 28.8246)
  line L67 (8.75, 11.5877) -> (8.75, 8.4123)
  line L68 (8.75, 30.4123) -> (6, 28.8246)
  line L69 (34.25, 11.5877) -> (37, 13.1754)
  line L70 (3.25, 30.4123) -> (3.25, 33.5877)
  line L71 (34.25, 30.4123) -> (34.25, 33.5877)
  line L72 (8.75, 8.4123) -> (6, 6.8246)
  line L73 (3.25, 33.5877) -> (6, 35.1754)
  line L74 (6, 6.8246) -> (3.25, 8.4123)
  line L75 (39.75, 33.5877) -> (39.75, 30.4123)
  line L76 (6, 28.8246) -> (3.25, 30.4123)
  line L77 (3.25, 11.5877) -> (6, 13.1754)
  line L78 (191.25, 8.4123) -> (194, 6.8246)
  line L79 (165.75, 11.5877) -> (163, 13.1754)
  line L80 (194, 6.8246) -> (196.75, 8.4123)
  line L81 (165.75, 30.4123) -> (165.75, 33.5877)
  line L82 (163, 28.8246) -> (165.75, 30.4123)
  line L83 (196.75, 11.5877) -> (194, 13.1754)
  line L84 (191.25, 30.4123) -> (194, 28.8246)
  line L85 (194, 13.1754) -> (191.25, 11.5877)
  line L86 (196.75, 33.5877) -> (194, 35.1754)
  line L87 (165.75, 33.5877) -> (163, 35.1754)
  line L88 (194, 35.1754) -> (191.25, 33.5877)
  line L89 (165.75, 8.4123) -> (165.75, 11.5877)
  line L90 (160.25, 11.5877) -> (160.25, 8.4123)
  line L91 (196.75, 30.4123) -> (196.75, 33.5877)
  line L92 (163, 6.8246) -> (165.75, 8.4123)
  line L93 (160.25, 33.5877) -> (160.25, 30.4123)
  line L94 (163, 13.1754) -> (160.25, 11.5877)
  line L95 (191.25, 11.5877) -> (191.25, 8.4123)
  line L96 (196.75, 8.4123) -> (196.75, 11.5877)
  line L97 (160.25, 30.4123) -> (163, 28.8246)
  line L98 (160.25, 8.4123) -> (163, 6.8246)
  line L99 (191.25, 33.5877) -> (191.25, 30.4123)
  line L100 (163, 35.1754) -> (160.25, 33.5877)
  line L101 (194, 28.8246) -> (196.75, 30.4123)
  point P0 (37, 240)
  point P1 (6, 240)
  point P2 (37, 218)
  point P3 (6, 218)
  point P4 (194, 240)
  point P5 (163, 218)
  point P6 (163, 218)
  point P7 (194, 240)
  point P8 (194, 218)
  point P9 (6, 10)
  point P10 (37, 10)
  point P11 (37, 10)
  point P12 (6, 32)
  point P13 (6, 10)
  point P14 (6, 32)
  point P15 (37, 32)
  point P16 (37, 32)
  point P17 (194, 10)
  point P18 (163, 10)
  point P19 (194, 32)
  point P20 (163, 32)
  point P21 (163, 32)
  point P22 (194, 32)
  point P23 (194, 10)
  point P24 (163, 32)
  point P25 (194, 10)
  dimension "d1" = 200
  dimension "d2" = 250
  dimension "d3" = 3
  dimension "d4" = 6
  dimension "d5" = 10
  dimension "d6" = 3
  dimension "d8" = 10
  dimension "d11" = 3
  dimension "d12" = 3
  dimension "d13" = 32
  dimension "d14" = 32
  dimension "d15" = 6
  dimension "d16" = 31
  dimension "d17" = 31
  dimension "d19" = 2.75
  dimension "d20" = 2.75
  dimension "d21" = 2.75
  dimension "d22" = 2.75
  constraint horizontal L0
  constraint vertical L1
  constraint horizontal L2
  constraint vertical L3
  constraint coincident L0.start L3.end
  constraint midpoint L2 L4.start
  constraint midpoint L0 L4.end
  constraint midpoint L3 L5.start
  constraint midpoint L1 L5.end
  constraint symmetric A0 L4 A3
  constraint symmetric A1 L4 A2
  constraint symmetric A0 L5 A4
  constraint symmetric A1 L5 A6
  constraint symmetric L5 A2 A5
  constraint symmetric L5 A3 A7
  constraint symmetric L4 A8 A11
  constraint symmetric L4 A9 A10
  constraint symmetric L5 A8 A13
  constraint symmetric L5 A9 A12
  constraint symmetric L5 A10 A15
  constraint symmetric L5 A11 A14
  constraint coincident P0 A1.centre
  constraint coincident P1 A0.centre
  constraint coincident P2 A9.centre
  constraint coincident P3 A8.centre
  constraint parallel L3 L15
  constraint parallel L11 L12
  constraint parallel L18 L27
  constraint parallel L3 L24
  constraint symmetric P1 L4 P7
  constraint symmetric L4 P2 P6
  constraint symmetric L4 L6.start L50.start
  constraint symmetric L4 L6.end L34.start
  constraint symmetric L4 L7.end L34.end
  constraint symmetric L4 L8.end L39.end
  constraint symmetric L4 L9.end L43.end
  constraint symmetric L4 L10.end L52.end
  constraint symmetric L4 L12.start L30.start
  constraint symmetric L4 L12.end L30.end
  constraint symmetric L4 L13.end L48.start
  constraint symmetric L4 L14.end L45.start
  constraint symmetric L4 L15.end L41.start
  constraint symmetric L4 L16.end L38.start
  constraint symmetric L4 P1 P7
  constraint symmetric L4 L18.start L44.start
  constraint symmetric L4 L18.end L44.end
  constraint symmetric L4 L19.end L33.start
  constraint symmetric L4 L20.end L33.end
  constraint symmetric L4 L21.end L32.start
  constraint symmetric L4 L22.end L32.end
  constraint symmetric L4 L24.start L35.end
  constraint symmetric L4 L24.end L37.end
  constraint symmetric L4 L25.end L31.start
  constraint symmetric L4 L26.end L31.end
  constraint symmetric L4 L27.end L36.start
  constraint symmetric L4 L28.end L35.start
  constraint symmetric L4 P3 P8
  constraint symmetric P1 L5 P13
  constraint symmetric P0 L5 P11
  constraint symmetric L5 P7 P25
  constraint symmetric L5 A2.centre P18
  constraint symmetric L5 P3 P14
  constraint symmetric L5 P2 P16
  constraint symmetric L5 P6 P24
  constraint symmetric L5 P8 P22
  constraint symmetric L5 L6.start L56.end
  constraint symmetric L5 L6.end L64.start
  constraint symmetric L5 L7.end L62.start
  constraint symmetric L5 L8.end L62.end
  constraint symmetric L5 L9.end L60.start
  constraint symmetric L5 L10.end L56.start
  constraint symmetric L5 P0 P11
  constraint symmetric L5 L12.start L63.end
  constraint symmetric L5 L12.end L67.end
  constraint symmetric L5 L13.end L72.end
  constraint symmetric L5 L14.end L61.start
  constraint symmetric L5 L15.end L61.end
  constraint symmetric L5 L16.end L63.start
  constraint symmetric L5 P1 P13
  constraint symmetric L5 L18.start L55.end
  constraint symmetric L5 L18.end L59.start
  constraint symmetric L5 L19.end L57.start
  constraint symmetric L5 L20.end L57.end
  constraint symmetric L5 L21.end L66.start
  constraint symmetric L5 L22.end L55.start
  constraint symmetric L5 L24.start L70.start
  constraint symmetric L5 L24.end L70.end
  constraint symmetric L5 L25.end L58.start
  constraint symmetric L5 L26.end L54.start
  constraint symmetric L5 L27.end L54.end
  constraint symmetric L5 L28.end L68.end
  constraint symmetric L5 L35.start L84.end
  constraint symmetric L5 L36.start L84.start
  constraint symmetric L5 L31.end L88.end
  constraint symmetric L5 L32.end L82.start
  constraint symmetric L5 L32.start L93.end
  constraint symmetric L5 L43.end L92.start
  constraint symmetric L5 L30.start L85.end
  constraint symmetric L5 L34.start L79.end
  constraint symmetric L5 L52.end L89.start
  constraint symmetric L5 L33.start L87.end
  constraint symmetric L5 L38.start L83.end
  constraint symmetric L5 L30.end L78.start
  constraint symmetric L5 L44.start L81.start
  constraint symmetric L5 L33.end L93.start
  constraint symmetric L5 L48.start L78.end
  constraint symmetric L5 L44.end L81.end
  constraint symmetric L5 L34.end L90.start
  constraint symmetric L5 L39.end L90.end
  constraint symmetric L5 L50.start L79.start
  constraint symmetric L5 L31.start L86.end
  constraint symmetric L5 L35.end L91.start
  constraint symmetric L5 L37.end L86.start
  constraint symmetric L5 L41.start L83.start
  constraint symmetric L5 L45.start L80.end
  measures "d1" distance of L0.start L0.end
  measures "d2" distance of L0.start L2.end
  measures "d3" diameter of A0
  measures "d4" distance of L3 P1
  measures "d5" distance of L2 P1
  measures "d6" diameter of A1
  measures "d8" distance of L2 P0
  measures "d11" diameter of A8
  measures "d12" diameter of A9
  measures "d13" distance of L2 P3
  measures "d14" distance of L2 P2
  measures "d15" distance of L3 P3
  measures "d16" distance of P1 P0
  measures "d17" distance of P3 P2
  measures "d19" distance of P0 L11
  measures "d20" distance of P1 L17
  measures "d21" distance of P2 L23
  measures "d22" distance of P3 L29
extrude "Extrude1" add sketch "Sketch1" along normal blind 5 contours L0 L3 L4 L5 | L0 L1 L4 L5 | L2 L3 L4 L5 | L1 L2 L4 L5 | L6 L7 L8 L9 L10 L11 | L12 L13 L14 L15 L16 L17 | L18 L19 L20 L21 L22 L23 | L24 L25 L26 L27 L28 L29 | L30 L38 L41 L45 L48 L51 | L31 L35 L36 L37 L42 L49 | L32 L33 L40 L44 L46 L47 | L34 L39 L43 L50 L52 L53 | L54 L58 L68 L70 L73 L76 | L55 L57 L59 L66 L71 L75 | L56 L60 L62 L64 L65 L69 | L61 L63 L67 L72 L74 L77 | L78 L80 L83 L85 L95 L96 | L79 L89 L90 L92 L94 L98 | L81 L82 L87 L93 L97 L100 | L84 L86 L88 L91 L99 L101
extrude "Extrude2" cut sketch "Sketch1" along normal blind 2.4 contours A12 | A13 | L6 L7 L8 L9 L10 L11 | L12 L13 L14 L15 L16 L17 | L18 L19 L20 L21 L22 L23 | L24 L25 L26 L27 L28 L29 | L30 L38 L41 L45 L48 L51 | L31 L35 L36 L37 L42 L49 | L32 L33 L40 L44 L46 L47 | L34 L39 L43 L50 L52 L53 | L54 L58 L68 L70 L73 L76 | L55 L57 L59 L66 L71 L75 | L56 L60 L62 L64 L65 L69 | L61 L63 L67 L72 L74 L77 | L78 L80 L83 L85 L95 L96 | L79 L89 L90 L92 L94 L98 | L81 L82 L87 L93 L97 L100 | L84 L86 L88 L91 L99 L101